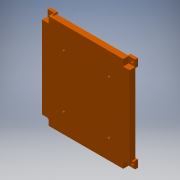
# Autodesk Inventor part: akksi-raspi
Saved by Autodesk Inventor 2019 (Build 230136000, 136)
## iProperties
Created: 2019-02-13
Part Number: akksi-raspi
Material: Generic
Document SubType Name: Modeling
Designer: izsoandras
Density: 1 g/cm^3
Appearance: Default
Author: izsoandras
Autodesk Inventor part; units mm, degrees
ref_plane "YZ Plane" through (0, 0, 0) normal (1, 0, 0) x (0, 1, 0)
ref_plane "XZ Plane" through (0, 0, 0) normal (0, 1, 0) x (-1, 0, 0)
ref_plane "XY Plane" through (0, 0, 0) normal (0, 0, 1) x (1, 0, 0)
sketch "Sketch1" plane through (0, 0, 0) normal (0, 0, 1) x (1, 0, 0)
  line L0 (47.0185, 51.5544) -> (-48.0003, 51.5544)
  line L1 (-48.0003, 51.5544) -> (-48.0003, -51.5544)
  line L2 (-48.0003, -51.5544) -> (47.0185, -51.5544)
  line L3 (47.0185, -51.5544) -> (47.0185, 51.5544)
  line L4 (41.2041, -35.74) -> (41.2041, 35.74) projected
  arc A0 (41.2041, 35.74) -> (31.2041, 45.74) centre (31.2041, 35.74) ccw projected
  line L5 (31.2041, 45.74) -> (-32.1859, 45.74) projected
  arc A1 (-32.1859, 45.74) -> (-42.1859, 35.74) centre (-32.1859, 35.74) ccw projected
  line L6 (-42.1859, 35.74) -> (-42.1859, -35.74) projected
  arc A2 (-42.1859, -35.74) -> (-32.1859, -45.74) centre (-32.1859, -35.74) ccw projected
  line L7 (-32.1859, -45.74) -> (31.2041, -45.74) projected
  arc A3 (31.2041, -45.74) -> (41.2041, -35.74) centre (31.2041, -35.74) ccw projected
  circle A4 centre (24.0591, 16.9245) radius 1.25 projected
  circle A5 centre (24.0591, -43.0755) radius 1.25 projected
  circle A6 centre (-25.0409, -43.0755) radius 1.25 projected
  circle A7 centre (-25.0409, 16.9245) radius 1.25 projected
  line L8 (25.5091, 38.0745) -> (-26.4909, 38.0745) projected
  arc A8 (-26.4909, 38.0745) -> (-28.4909, 36.0745) centre (-26.4909, 36.0745) ccw projected
  line L9 (-28.4909, 36.0745) -> (-28.4909, -44.9255) projected
  arc A9 (-28.4909, -44.9255) -> (-26.4909, -46.9255) centre (-26.4909, -44.9255) ccw projected
  line L10 (-26.4909, -46.9255) -> (25.5091, -46.9255) projected
  arc A10 (25.5091, -46.9255) -> (27.5091, -44.9255) centre (25.5091, -44.9255) ccw projected
  line L11 (27.5091, -44.9255) -> (27.5091, 36.0745) projected
  arc A11 (27.5091, 36.0745) -> (25.5091, 38.0745) centre (25.5091, 36.0745) ccw projected
  point P0 (0, 0)
  dimension "d2" = 5.8144
  dimension "d3" = 5.8144
  dimension "d4" = 5.8144
  dimension "d5" = 5.8144
  constraints: 8 end point, 2 parallel, 1 horizontal, 1 perpendicular
  measures "d2" distance between parallel lines of L3 L4
  measures "d3" distance between parallel lines of L6 L1
  measures "d4" distance between parallel lines of L0 L5
  measures "d5" distance between parallel lines of L2 L7
extrude "Extrusion1" add sketch "Sketch1" along normal blind 3 contours L3 L2 L1 L0 | A3 L7 A10 L11 A11 L8 A8 L9 A9 A2 L6 A1 L5 A0 L4 | A10 L10 A9 L7 | L7 A9 L9 A8 L8 A11 L11 A10 | A4 | A5 | A6 | A7
sketch "Sketch3" plane through (0, 0, 0) normal (0, 0, -1) x (-1, 0, 0)
  line L0 (-41.2041, 35.74) -> (-41.2041, -35.74) projected
  arc A0 (-41.2041, -35.74) -> (-31.2041, -45.74) centre (-31.2041, -35.74) ccw projected
  line L1 (-31.2041, -45.74) -> (32.1859, -45.74) projected
  arc A1 (32.1859, -45.74) -> (42.1859, -35.74) centre (32.1859, -35.74) ccw projected
  line L2 (42.1859, -35.74) -> (42.1859, 35.74) projected
  arc A2 (42.1859, 35.74) -> (32.1859, 45.74) centre (32.1859, 35.74) ccw projected
  line L3 (32.1859, 45.74) -> (-31.2041, 45.74) projected
  arc A3 (-31.2041, 45.74) -> (-41.2041, 35.74) centre (-31.2041, 35.74) ccw projected
  line L4 (43.1859, 43.5544) -> (46.1859, 43.5544)
  line L5 (46.1859, 43.5544) -> (46.1859, -43.5544)
  line L6 (46.1859, -43.5544) -> (43.1859, -43.5544)
  line L7 (43.1859, -43.5544) -> (43.1859, 43.5544)
  line L8 (-42.2041, 43.5544) -> (-45.2041, 43.5544)
  line L9 (-45.2041, 43.5544) -> (-45.2041, -43.5544)
  line L10 (-45.2041, -43.5544) -> (-42.2041, -43.5544)
  line L11 (-42.2041, -43.5544) -> (-42.2041, 43.5544)
  line L12 (40.0003, 49.74) -> (-39.0185, 49.74)
  line L13 (-39.0185, 49.74) -> (-39.0185, 46.74)
  line L14 (-39.0185, 46.74) -> (40.0003, 46.74)
  line L15 (40.0003, 46.74) -> (40.0003, 49.74)
  line L16 (40.0003, -46.74) -> (-39.0185, -46.74)
  line L17 (-39.0185, -46.74) -> (-39.0185, -49.74)
  line L18 (-39.0185, -49.74) -> (40.0003, -49.74)
  line L19 (40.0003, -49.74) -> (40.0003, -46.74)
  line L20 (-47.0185, 51.5544) -> (48.0003, 51.5544) projected
  line L21 (48.0003, 51.5544) -> (48.0003, -51.5544) projected
  line L22 (48.0003, -51.5544) -> (-47.0185, -51.5544) projected
  line L23 (-47.0185, -51.5544) -> (-47.0185, 51.5544) projected
  point P0 (0, 0)
  dimension "d20" = 3
  dimension "d21" = 1
  dimension "d24" = 3
  dimension "d25" = 1
  dimension "d28" = 3
  dimension "d29" = 1
  dimension "d34" = 1
  dimension "d35" = 3
  dimension "d78" = 8
  dimension "d79" = 8
  dimension "d80" = 8
  dimension "d81" = 8
  dimension "d82" = 8
  dimension "d83" = 8
  dimension "d84" = 8
  dimension "d85" = 8
  constraints: 32 end point, 8 parallel, 4 horizontal, 4 perpendicular, 1 other
  measures "d20" distance of L5.end L6.end
  measures "d21" distance between parallel lines of L2 L7
  measures "d24" distance of L8.start L8.end
  measures "d25" distance between parallel lines of L0 L11
  measures "d28" distance of L14.end L12.start
  measures "d29" distance between parallel lines of L3 L14
  measures "d34" distance between parallel lines of L16 L1
  measures "d35" distance of L18.end L16.start
  measures "d78" distance between parallel lines of L20 L4
  measures "d79" distance between parallel lines of L21 L15
  measures "d80" distance between parallel lines of L22 L6
  measures "d81" distance between parallel lines of L21 L19
  measures "d82" distance between parallel lines of L23 L17
  measures "d83" distance between parallel lines of L22 L10
  measures "d84" distance between parallel lines of L20 L8
  measures "d85" distance between parallel lines of L23 L13
extrude "Extrusion2" add sketch "Sketch3" along normal blind 5 contours L4 L5 L6 L7 | L11 L10 L9 L8 | L15 L14 L13 L12 | L19 L18 L17 L16
sketch "Sketch6" plane through (0, 0, 0) normal (0, 0, -1) x (-1, 0, 0)
  line L0 (48.0003, 51.5544) -> (48.0003, -51.5544) projected
  line L1 (48.0003, 51.5544) -> (40.0003, 51.5544)
  line L2 (40.0003, 51.5544) -> (40.0003, 43.5544)
  line L3 (40.0003, 43.5544) -> (48.0003, 43.5544)
  line L4 (48.0003, 43.5544) -> (48.0003, 51.5544)
  line L5 (48.0003, -51.5544) -> (40.0003, -51.5544)
  line L6 (40.0003, -51.5544) -> (40.0003, -43.5544)
  line L7 (40.0003, -43.5544) -> (48.0003, -43.5544)
  line L8 (48.0003, -43.5544) -> (48.0003, -51.5544)
  line L9 (48.0003, -51.5544) -> (-47.0185, -51.5544) projected
  line L10 (-47.0185, -51.5544) -> (-39.0185, -51.5544)
  line L11 (-39.0185, -51.5544) -> (-39.0185, -43.5544)
  line L12 (-39.0185, -43.5544) -> (-47.0185, -43.5544)
  line L13 (-47.0185, -43.5544) -> (-47.0185, -51.5544)
  line L14 (-47.0185, 51.5544) -> (48.0003, 51.5544) projected
  line L15 (-47.0185, 51.5544) -> (-39.0185, 51.5544)
  line L16 (-39.0185, 51.5544) -> (-39.0185, 43.5544)
  line L17 (-39.0185, 43.5544) -> (-47.0185, 43.5544)
  line L18 (-47.0185, 43.5544) -> (-47.0185, 51.5544)
  point P0 (0, 0)
  dimension "d38" = 8
  dimension "d39" = 8
  dimension "d40" = 8
  dimension "d41" = 8
  dimension "d42" = 8
  dimension "d43" = 8
  dimension "d44" = 8
  dimension "d45" = 8
  constraints: 32 end point, 8 parallel, 4 horizontal, 4 perpendicular
  measures "d38" distance of L2.end L3.end
  measures "d39" distance of L1.end L2.end
  measures "d40" distance of L15.end L16.end
  measures "d41" distance of L16.end L17.end
  measures "d42" distance of L11.end L12.end
  measures "d43" distance of L12.end L9.end
  measures "d44" distance of L6.end L7.end
  measures "d45" distance of L5.end L6.end
extrude "Extrusion3" add sketch "Sketch6" along normal blind 6
sketch "Sketch7" plane through (0, 0, 3) normal (0, 0, 1) x (1, 0, 0)
  line L0 (47.0185, -51.5544) -> (47.0185, 51.5544) projected
  line L1 (47.0185, 51.5544) -> (40.0185, 51.5544)
  line L2 (40.0185, 51.5544) -> (40.0185, 44.5544)
  line L3 (40.0185, 44.5544) -> (47.0185, 44.5544)
  line L4 (47.0185, 44.5544) -> (47.0185, 51.5544)
  line L5 (47.0185, -51.5544) -> (40.0185, -51.5544)
  line L6 (40.0185, -51.5544) -> (40.0185, -44.5544)
  line L7 (40.0185, -44.5544) -> (47.0185, -44.5544)
  line L8 (47.0185, -44.5544) -> (47.0185, -51.5544)
  line L9 (-48.0003, 51.5544) -> (-48.0003, -51.5544) projected
  line L10 (-48.0003, -51.5544) -> (-41.0003, -51.5544)
  line L11 (-41.0003, -51.5544) -> (-41.0003, -44.5544)
  line L12 (-41.0003, -44.5544) -> (-48.0003, -44.5544)
  line L13 (-48.0003, -44.5544) -> (-48.0003, -51.5544)
  line L14 (-48.0003, 51.5544) -> (-41.0003, 51.5544)
  line L15 (-41.0003, 51.5544) -> (-41.0003, 44.5544)
  line L16 (-41.0003, 44.5544) -> (-48.0003, 44.5544)
  line L17 (-48.0003, 44.5544) -> (-48.0003, 51.5544)
  point P0 (0, 0)
  dimension "d48" = 7
  dimension "d49" = 7
  dimension "d50" = 7
  dimension "d51" = 7
  dimension "d52" = 7
  dimension "d53" = 7
  dimension "d54" = 7
  dimension "d55" = 7
  constraints: 32 end point, 8 parallel, 4 horizontal, 4 perpendicular
  measures "d48" distance of L2.end L3.end
  measures "d49" distance of L1.end L2.end
  measures "d50" distance of L6.end L7.end
  measures "d51" distance of L5.end L6.end
  measures "d52" distance of L14.end L15.end
  measures "d53" distance of L15.end L16.end
  measures "d54" distance of L10.end L11.end
  measures "d55" distance of L11.end L12.end
extrude "Extrusion4" cut sketch "Sketch7" against normal blind 6
sketch "Sketch8" plane through (0, 0, -3) normal (0, 0, 1) x (1, 0, 0)
  circle A0 centre (43.5185, 48.0544) radius 1.5
  circle A1 centre (43.5185, -48.0544) radius 1.5
  circle A2 centre (-44.5003, -48.0544) radius 1.5
  circle A3 centre (-44.5003, 48.0544) radius 1.5
  line L0 (47.0185, 51.5544) -> (47.0185, 44.5544) projected
  line L1 (40.0185, 51.5544) -> (47.0185, 51.5544) projected
  line L2 (47.0185, -44.5544) -> (47.0185, -51.5544) projected
  line L3 (47.0185, -51.5544) -> (40.0185, -51.5544) projected
  line L4 (-48.0003, -51.5544) -> (-48.0003, -44.5544) projected
  line L5 (-41.0003, -51.5544) -> (-48.0003, -51.5544) projected
  line L6 (-48.0003, 44.5544) -> (-48.0003, 51.5544) projected
  line L7 (-48.0003, 51.5544) -> (-41.0003, 51.5544) projected
  point P0 (0, 0)
  dimension "d58" = 3
  dimension "d59" = 3
  dimension "d60" = 3
  dimension "d61" = 3
  dimension "d62" = 3.5
  dimension "d63" = 3.5
  dimension "d64" = 3.5
  dimension "d65" = 3.5
  dimension "d66" = 3.5
  dimension "d67" = 3.5
  dimension "d68" = 3.5
  dimension "d69" = 3.5
  constraints: 4 centre point
  measures "d58" diameter of A0
  measures "d59" diameter of A1
  measures "d60" diameter of A2
  measures "d61" diameter of A3
  measures "d62" distance from line of L0 A0.centre
  measures "d63" distance from line of L1 A0.centre
  measures "d64" distance from line of L2 A1.centre
  measures "d65" distance from line of L3 A1.centre
  measures "d66" distance from line of L4 A2.centre
  measures "d67" distance from line of L5 A2.centre
  measures "d68" distance from line of L6 A3.centre
  measures "d69" distance from line of L7 A3.centre
extrude "Extrusion5" cut sketch "Sketch8" against normal up to next
sketch "Sketch9" plane through (0, 0, 3) normal (0, 0, 1) x (1, 0, 0)
  circle A0 centre (24.0497, -29.5956) radius 1.25 projected
  circle A1 centre (-25.0503, -29.5956) radius 1.25 projected
  line L0 (25.4997, 51.5544) -> (-26.5003, 51.5544) projected
  arc A2 (-26.5003, 51.5544) -> (-28.5003, 49.5544) centre (-26.5003, 49.5544) ccw projected
  line L1 (-28.5003, 49.5544) -> (-28.5003, -31.4456) projected
  arc A3 (-28.5003, -31.4456) -> (-26.5003, -33.4456) centre (-26.5003, -31.4456) ccw projected
  line L2 (-26.5003, -33.4456) -> (25.4997, -33.4456) projected
  arc A4 (25.4997, -33.4456) -> (27.4997, -31.4456) centre (25.4997, -31.4456) ccw projected
  line L3 (27.4997, -31.4456) -> (27.4997, 49.5544) projected
  arc A5 (27.4997, 49.5544) -> (25.4997, 51.5544) centre (25.4997, 49.5544) ccw projected
  circle A6 centre (24.0497, -29.5956) radius 1.5
  circle A7 centre (-25.0503, -29.5956) radius 1.5
  circle A8 centre (24.0497, 27.9044) radius 1.25 projected
  circle A9 centre (24.0497, -29.5956) radius 1.25 projected
  circle A10 centre (-25.0503, -29.5956) radius 1.25 projected
  circle A11 centre (-25.0503, 27.9044) radius 1.25 projected
  line L4 (25.4997, 51.5544) -> (-26.5003, 51.5544) projected
  arc A12 (-26.5003, 51.5544) -> (-28.5003, 49.5544) centre (-26.5003, 49.5544) ccw projected
  line L5 (-28.5003, 49.5544) -> (-28.5003, -31.4456) projected
  arc A13 (-28.5003, -31.4456) -> (-26.5003, -33.4456) centre (-26.5003, -31.4456) ccw projected
  line L6 (-26.5003, -33.4456) -> (25.4997, -33.4456) projected
  arc A14 (25.4997, -33.4456) -> (27.4997, -31.4456) centre (25.4997, -31.4456) ccw projected
  line L7 (27.4997, -31.4456) -> (27.4997, 49.5544) projected
  arc A15 (27.4997, 49.5544) -> (25.4997, 51.5544) centre (25.4997, 49.5544) ccw projected
  circle A16 centre (24.0497, 27.9044) radius 1.5
  circle A17 centre (-25.0503, 27.9044) radius 1.5
  point P0 (0, 0)
  dimension "d73" = 3
  dimension "d74" = 3
  dimension "d86" = 3
  dimension "d87" = 3
  constraints: 4 centre point, 4 coincident
  measures "d73" diameter of A6
  measures "d74" diameter of A7
  measures "d86" diameter of A16
  measures "d87" diameter of A17
extrude "Extrusion6" cut sketch "Sketch9" against normal up to next contours A0 | A1 | A6 | A7 | A8 | A11 | A16 | A17
equation "\"d3\" = d2"
equation "\"d4\" = d2"
equation "\"d5\" = d2"
equation "\"d39\" = d38"
equation "\"d40\" = d38"
equation "\"d41\" = d38"
equation "\"d42\" = d38"
equation "\"d43\" = d38"
equation "\"d44\" = d38"
equation "\"d45\" = d38"
equation "\"d49\" = d48"
equation "\"d50\" = d48"
equation "\"d51\" = d48"
equation "\"d52\" = d48"
equation "\"d53\" = d48"
equation "\"d54\" = d48"
equation "\"d55\" = d48"
equation "\"d62\" = 0.5 * d48"
equation "\"d63\" = d62"
equation "\"d64\" = d62"
equation "\"d65\" = d62"
equation "\"d66\" = d62"
equation "\"d67\" = d62"
equation "\"d68\" = d62"
equation "\"d69\" = d62"
equation "\"d74\" = d73"
equation "\"d86\" = d73"
equation "\"d87\" = d73"
body "Solid1"
